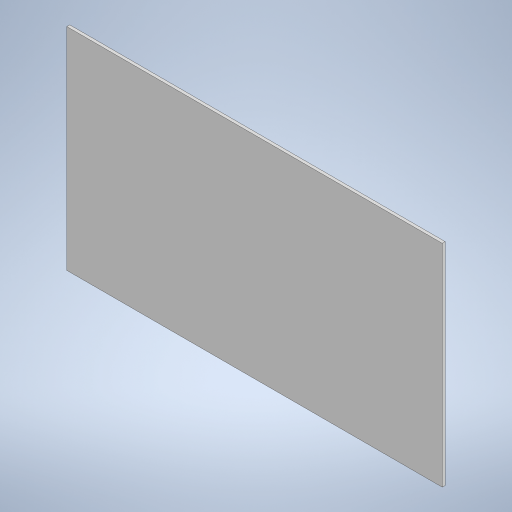
# Autodesk Inventor part: top_plywood_Ocampo
Saved by Autodesk Inventor 2023 (Build 270158000, 158)
## iProperties
Created: 2025-02-18
Part Number: top_plywood_Ocampo
Material: Generic
Document SubType Name: Modeling
Designer: 1244275
Density: 1 g/cm^3
Appearance: Default
Author: 1244275
Autodesk Inventor part; units mm, degrees
ref_plane "YZ Plane" through (0, 0, 0) normal (1, 0, 0) x (0, 1, 0)
ref_plane "XZ Plane" through (0, 0, 0) normal (0, 1, 0) x (-1, 0, 0)
ref_plane "XY Plane" through (0, 0, 0) normal (0, 0, 1) x (1, 0, 0)
sketch "Sketch1" plane through (0, 0, 0) normal (0, 0, 1) x (1, 0, 0)
  line L0 (0, 0) -> (0, 457.2)
  line L1 (0, 457.2) -> (812.8, 457.2)
  line L2 (812.8, 457.2) -> (812.8, 0)
  line L3 (812.8, 0) -> (0, 0)
  line L4 (0, 0) -> (812.8, 0)
  dimension "d0" = 457.2
  dimension "d1" = 812.8
  constraints: 10 end point, 3 perpendicular, 1 horizontal, 1 vertical
  measures "d0" distance of L0.start L0.end
  measures "d1" distance of L0.end L1.end
extrude "Extrusion1" add sketch "Sketch1" along normal blind 6.35
body "Solid1"
